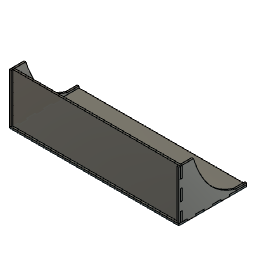
Hilla (Autodesk Fusion 360 design; units mm, degrees)
Autodesk Fusion 360 part; units mm, degrees
sketch "Sketch1" plane through (0, 0, 0) normal (0, 1, 0) x (1, 0, 0)
sketch "Sketch2" plane through (0, 0, 0) normal (0, 1, 0) x (1, 0, 0)
  line L0 (0, 0) -> (500, 0)
  line L1 (500, 0) -> (500, 200)
  line L2 (500, 200) -> (0, 200)
  line L3 (0, 200) -> (0, 0)
  dimension "d5" = 200
  dimension "d6" = 500
  constraint horizontal L0
  constraint vertical L1
  constraint horizontal L2
  constraint vertical L3
  constraint coincident L0.start L3.end
  measures "d5" distance of L0.start L2.end
  measures "d6" distance of L0.start L0.end
extrude "Extrude1" add sketch "Sketch2" along normal blind 5 makes body 1
sketch "Sketch3" plane through (0, 5, 0) normal (0, 1, 0) x (-1, 0, 0)
  line L0 (0, -200) -> (0, 0)
  line L1 (0, 0) -> (-500, 0)
  line L2 (-500, 0) -> (-500, -200)
  line L3 (-500, -200) -> (0, -200)
  line L4 (0, 0) -> (0, -25)
  line L5 (0, -25) -> (-5, -25)
  line L6 (-5, -25) -> (-5, -50)
  line L7 (-5, -50) -> (0, -50)
  line L8 (0, -50) -> (0, -25)
  dimension "d9" = 25
  dimension "d10" = 5
  dimension "d11" = 25
  constraint vertical L4
  constraint coincident L0.end L1.start
  constraint horizontal L5
  constraint vertical L6
  constraint horizontal L7
  constraint vertical L8
  measures "d9" distance of L0.end L4.end
  measures "d10" distance of L4.end L5.end
  measures "d11" distance of L4.end L7.end
extrude "Extrude2" cut sketch "Sketch3" against normal blind 5 contours L0 L5 L6 L7 L8 bodies 1
sketch "Sketch4" plane through (0, 5, 0) normal (0, 1, 0) x (-1, 0, 0)
  line L0 (-5, -25) -> (0, -25)
  line L1 (0, -25) -> (0, 0)
  line L2 (0, 0) -> (-500, 0)
  line L3 (-500, 0) -> (-500, -200)
  line L4 (-500, -200) -> (0, -200)
  line L5 (0, -200) -> (0, -50)
  line L6 (0, -50) -> (-5, -50)
  line L7 (-5, -50) -> (-5, -25)
  line L8 (0, -50) -> (0, -75)
  line L9 (0, -75) -> (-5, -75)
  line L10 (-5, -75) -> (-5, -100)
  line L11 (-5, -100) -> (0, -100)
  line L12 (0, -100) -> (0, -75)
  line L13 (0, -100) -> (0, -125)
  line L14 (0, -125) -> (-5, -125)
  line L15 (-5, -125) -> (-5, -150)
  line L16 (-5, -150) -> (0, -150)
  line L17 (0, -150) -> (0, -125)
  dimension "d14" = 25
  dimension "d15" = 5
  dimension "d16" = 25
  dimension "d17" = 25
  dimension "d18" = 25
  dimension "d19" = 5
  constraint vertical L8
  constraint coincident L5.end L6.start
  constraint horizontal L9
  constraint vertical L10
  constraint horizontal L11
  constraint vertical L12
  constraint vertical L13
  constraint horizontal L14
  constraint vertical L15
  constraint horizontal L16
  constraint vertical L17
  measures "d14" distance of L5.end L8.end
  measures "d15" distance of L8.end L9.end
  measures "d16" distance of L8.end L11.end
  measures "d17" distance of L11.end L13.end
  measures "d18" distance of L13.end L16.end
  measures "d19" distance of L13.end L14.end
extrude "Extrude3" cut sketch "Sketch4" against normal blind 5 contours L5 L9 L10 L11 L12 | L5 L14 L15 L16 L17 bodies 1
sketch "Sketch5" plane through (0, 5, 0) normal (0, 1, 0) x (-1, 0, 0)
  line L0 (0, -150) -> (-5, -150)
  line L1 (-5, -150) -> (-5, -125)
  line L2 (-5, -125) -> (0, -125)
  line L3 (0, -125) -> (0, -100)
  line L4 (0, -100) -> (-5, -100)
  line L5 (-5, -100) -> (-5, -75)
  line L6 (-5, -75) -> (0, -75)
  line L7 (0, -75) -> (0, -50)
  line L8 (0, -50) -> (-5, -50)
  line L9 (-5, -50) -> (-5, -25)
  line L10 (-5, -25) -> (0, -25)
  line L11 (0, -25) -> (0, 0)
  line L12 (0, 0) -> (-500, 0)
  line L13 (-500, 0) -> (-500, -200)
  line L14 (-500, -200) -> (0, -200)
  line L15 (0, -200) -> (0, -150)
  line L16 (-500, 0) -> (-500, -25)
  line L17 (-500, -25) -> (-495, -25)
  line L18 (-495, -25) -> (-495, -50)
  line L19 (-495, -50) -> (-500, -50)
  line L20 (-500, -50) -> (-500, -25)
  line L21 (-500, -50) -> (-500, -37.5)
  line L22 (-500, -37.5) -> (-495, -37.5)
  line L23 (-495, -37.5) -> (-495, -62.5)
  line L24 (-495, -62.5) -> (-500, -62.5)
  line L25 (-500, -62.5) -> (-500, -37.5)
  line L26 (-500, -62.5) -> (-500, -87.5)
  line L27 (-500, -87.5) -> (-495, -87.5)
  line L28 (-495, -87.5) -> (-495, -112.5)
  line L29 (-495, -112.5) -> (-500, -112.5)
  line L30 (-500, -112.5) -> (-500, -87.5)
  dimension "d22" = 25
  dimension "d23" = 5
  dimension "d24" = 25
  dimension "d26" = 25
  dimension "d27" = 5
  dimension "d28" = 25
  dimension "d29" = 25
  dimension "d30" = 5
  constraint vertical L16
  constraint coincident L12.end L13.start
  constraint horizontal L17
  constraint vertical L18
  constraint horizontal L19
  constraint vertical L20
  constraint vertical L21
  constraint horizontal L22
  constraint vertical L23
  constraint horizontal L24
  constraint vertical L25
  constraint vertical L26
  constraint horizontal L27
  constraint vertical L28
  constraint horizontal L29
  constraint vertical L30
  measures "d22" distance of L12.end L16.end
  measures "d23" distance of L16.end L17.end
  measures "d24" distance of L16.end L19.end
  measures "d26" distance of L21.end L24.end
  measures "d27" distance of L21.end L22.end
  measures "d28" distance of L24.end L26.end
  measures "d29" distance of L26.end L29.end
  measures "d30" distance of L26.end L27.end
extrude "Extrude4" cut sketch "Sketch5" against normal blind 5 contours L13 L27 L28 L29 L30 | L13 L19 L23 L24 L25 | L13 L18 L19 L20 L21 L22 L23 L25 | L13 L17 L18 L20 L22 bodies 1
sketch "Sketch6" plane through (0, 5, 0) normal (0, 1, 0) x (-1, 0, 0)
  line L0 (-500, -87.5) -> (-495, -87.5)
  line L1 (-495, -87.5) -> (-495, -112.5)
  line L2 (-500, -62.5) -> (-500, -87.5)
  line L3 (-500, -200) -> (0, -200)
  line L4 (0, -200) -> (0, -150)
  line L5 (0, -150) -> (-5, -150)
  line L6 (-5, -150) -> (-5, -125)
  line L7 (-5, -125) -> (0, -125)
  line L8 (0, -125) -> (0, -100)
  line L9 (0, -100) -> (-5, -100)
  line L10 (-5, -100) -> (-5, -75)
  line L11 (-5, -75) -> (0, -75)
  line L12 (0, -75) -> (0, -50)
  line L13 (0, -50) -> (-5, -50)
  line L14 (-5, -50) -> (-5, -25)
  line L15 (-5, -25) -> (0, -25)
  line L16 (0, -25) -> (0, 0)
  line L17 (0, 0) -> (-500, 0)
  line L18 (-500, 0) -> (-500, -25)
  line L19 (0, 0) -> (0, -5)
  line L20 (0, -5) -> (-60, -5)
  line L21 (-60, -5) -> (-110, -5)
  line L22 (-110, -5) -> (-110, -10)
  line L23 (-110, -10) -> (-60, -10)
  line L24 (-60, -10) -> (-60, -5)
  line L25 (-110, -5) -> (-170, -5)
  line L26 (-170, -5) -> (-220, -5)
  line L27 (-220, -5) -> (-220, -10)
  line L28 (-220, -10) -> (-170, -10)
  line L29 (-170, -10) -> (-170, -5)
  line L30 (-220, -5) -> (-280, -5)
  line L31 (-280, -5) -> (-330, -5)
  line L32 (-330, -5) -> (-330, -10)
  line L33 (-330, -10) -> (-280, -10)
  line L34 (-280, -10) -> (-280, -5)
  line L35 (-330, -5) -> (-390, -5)
  line L36 (-390, -5) -> (-440, -5)
  line L37 (-440, -5) -> (-440, -10)
  line L38 (-440, -10) -> (-390, -10)
  line L39 (-390, -10) -> (-390, -5)
  line L40 (-500, -25) -> (-495, -25)
  line L41 (-495, -25) -> (-495, -62.5)
  line L42 (-495, -62.5) -> (-500, -62.5)
  line L43 (-495, -112.5) -> (-500, -112.5)
  line L44 (-500, -112.5) -> (-500, -200)
  dimension "d33" = 5
  dimension "d34" = 60
  dimension "d35" = 50
  dimension "d36" = 5
  dimension "d37" = 60
  dimension "d38" = 50
  dimension "d39" = 5
  dimension "d40" = 60
  dimension "d41" = 50
  dimension "d42" = 5
  dimension "d43" = 60
  dimension "d44" = 50
  dimension "d45" = 5
  constraint vertical L19
  constraint coincident L16.end L17.start
  constraint horizontal L20
  constraint horizontal L21
  constraint vertical L22
  constraint horizontal L23
  constraint vertical L24
  constraint horizontal L25
  constraint horizontal L26
  constraint vertical L27
  constraint horizontal L28
  constraint vertical L29
  constraint horizontal L30
  constraint horizontal L31
  constraint vertical L32
  constraint horizontal L33
  constraint vertical L34
  constraint horizontal L35
  constraint horizontal L36
  constraint vertical L37
  constraint horizontal L38
  constraint vertical L39
  measures "d33" distance of L16.end L19.end
  measures "d34" distance of L19.end L20.end
  measures "d35" distance of L20.end L21.end
  measures "d36" distance of L20.end L23.end
  measures "d37" distance of L21.end L25.end
  measures "d38" distance of L25.end L26.end
  measures "d39" distance of L25.end L28.end
  measures "d40" distance of L26.end L30.end
  measures "d41" distance of L30.end L31.end
  measures "d42" distance of L30.end L33.end
  measures "d43" distance of L31.end L35.end
  measures "d44" distance of L35.end L36.end
  measures "d45" distance of L35.end L38.end
extrude "Extrude5" cut sketch "Sketch6" against normal blind 5 contours L21 L22 L23 L24 | L26 L27 L28 L29 | L31 L32 L33 L34 | L36 L37 L38 L39 bodies 1
sketch "Sketch7" plane through (0, 0, -10) normal (0, 0, 1) x (1, 0, 0)
  line L0 (110, 5) -> (60, 5)
  line L1 (60, 5) -> (60, 0)
  line L2 (60, 0) -> (110, 0)
  line L3 (110, 0) -> (110, 5)
  line L4 (0, 0) -> (500, 0)
  line L5 (500, 0) -> (500, 150)
  line L6 (500, 150) -> (0, 150)
  line L7 (0, 150) -> (0, 0)
  dimension "d48" = 500
  dimension "d49" = 150
  constraint horizontal L4
  constraint vertical L5
  constraint horizontal L6
  constraint vertical L7
  constraint coincident L4.start L7.end
  measures "d48" distance of L4.start L4.end
  measures "d49" distance of L4.start L6.end
extrude "Extrude6" add sketch "Sketch7" along normal blind 5 separate body contours L0 L1 L3 L4 L5 L6 L7 makes body 2
sketch "Sketch8" plane through (0, 0, 0) normal (-1, 0, 0) x (0, 0, 1)
  line L0 (-10, 150) -> (-10, 0)
  line L1 (-10, 0) -> (-5, 0)
  line L2 (-5, 0) -> (-5, 150)
  line L3 (-5, 150) -> (-10, 150)
  line L4 (-5, 150) -> (-5, 116.6667)
  line L5 (-5, 116.6667) -> (-10, 116.6667)
  line L6 (-10, 116.6667) -> (-10, 91.6667)
  line L7 (-10, 91.6667) -> (-5, 91.6667)
  line L8 (-5, 91.6667) -> (-5, 116.6667)
  line L9 (-5, 91.6667) -> (-5, 58.3333)
  line L10 (-5, 58.3333) -> (-10, 58.3333)
  line L11 (-10, 58.3333) -> (-10, 33.3333)
  line L12 (-10, 33.3333) -> (-5, 33.3333)
  line L13 (-5, 33.3333) -> (-5, 58.3333)
  dimension "d52" = 33.3333
  dimension "d53" = 25
  dimension "d54" = 5
  dimension "d55" = 33.3333
  dimension "d56" = 25
  dimension "d57" = 5
  constraint vertical L4
  constraint coincident L2.end L3.start
  constraint horizontal L5
  constraint vertical L6
  constraint horizontal L7
  constraint vertical L8
  constraint vertical L9
  constraint horizontal L10
  constraint vertical L11
  constraint horizontal L12
  constraint vertical L13
  measures "d52" distance of L2.end L4.end
  measures "d53" distance of L4.end L7.end
  measures "d54" distance of L4.end L5.end
  measures "d55" distance of L7.end L9.end
  measures "d56" distance of L9.end L12.end
  measures "d57" distance of L9.end L10.end
extrude "Extrude7" cut sketch "Sketch8" against normal blind 5 contours L0 L2 L5 L6 L7 L8 | L0 L2 L10 L11 L12 L13 bodies 2
extrude "Extrude8" add 1 faces at (93.3333, 5, -8.3333) along direction (0, -1, 0) blind 5 on bodies 2 bodies 2
combine "Combine1" operation cut target body 2 tool bodies 1 keep tools
sketch "Sketch9" plane through (500, 0, 0) normal (1, 0, 0) x (0, 0, -1)
  line L0 (5, 5) -> (10, 5)
  line L1 (10, 5) -> (10, 150)
  line L2 (10, 150) -> (5, 150)
  line L3 (5, 150) -> (5, 5)
  line L4 (5, 150) -> (5, 116.6667)
  line L5 (5, 116.6667) -> (10, 116.6667)
  line L6 (10, 116.6667) -> (10, 91.6667)
  line L7 (10, 91.6667) -> (5, 91.6667)
  line L8 (5, 91.6667) -> (5, 116.6667)
  line L9 (5, 91.6667) -> (5, 58.3333)
  line L10 (5, 58.3333) -> (10, 58.3333)
  line L11 (10, 58.3333) -> (10, 33.3333)
  line L12 (10, 33.3333) -> (5, 33.3333)
  line L13 (5, 33.3333) -> (5, 58.3333)
  dimension "d62" = 33.3333
  dimension "d63" = 5
  dimension "d64" = 25
  dimension "d65" = 33.3333
  dimension "d66" = 5
  dimension "d67" = 25
  constraint vertical L4
  constraint coincident L2.end L3.start
  constraint horizontal L5
  constraint vertical L6
  constraint horizontal L7
  constraint vertical L8
  constraint vertical L9
  constraint horizontal L10
  constraint vertical L11
  constraint horizontal L12
  constraint vertical L13
  measures "d62" distance of L2.end L4.end
  measures "d63" distance of L4.end L5.end
  measures "d64" distance of L4.end L7.end
  measures "d65" distance of L7.end L9.end
  measures "d66" distance of L9.end L10.end
  measures "d67" distance of L9.end L12.end
extrude "Extrude9" cut sketch "Sketch9" against normal blind 5 contours L1 L3 L10 L11 L12 L13 | L1 L3 L5 L6 L7 L8 bodies 2
sketch "Sketch10" plane through (495, 0, 0) normal (1, 0, 0) x (0, 0, -1)
  line L0 (62.5, 5) -> (25, 5)
  line L1 (25, 0) -> (62.5, 0)
  line L2 (62.5, 0) -> (62.5, 5)
  line L3 (0, 0) -> (200, 0)
  line L4 (200, 0) -> (200, 150)
  line L5 (200, 150) -> (0, 150)
  line L6 (0, 150) -> (0, 0)
  line L7 (62.5, 5) -> (37.5, 5)
  line L8 (37.5, 5) -> (37.5, 0)
  line L9 (37.5, 0) -> (62.5, 0)
  line L10 (62.5, 0) -> (62.5, 5)
  line L11 (25, 5) -> (25, 0)
  dimension "d70" = 200
  dimension "d71" = 150
  dimension "d72" = 25
  dimension "d73" = 5
  constraint horizontal L3
  constraint vertical L4
  constraint horizontal L5
  constraint vertical L6
  constraint coincident L3.start L6.end
  constraint horizontal L7
  constraint vertical L8
  constraint horizontal L9
  constraint vertical L10
  constraint coincident L0.start L2.end
  measures "d70" distance of L3.start L3.end
  measures "d71" distance of L3.start L5.end
  measures "d72" distance of L0.start L7.end
  measures "d73" distance of L0.start L1.end
sketch "Sketch11" plane through (500, 0, 0) normal (1, 0, 0) x (0, 0, -1)
  line L0 (10, 58.3333) -> (5, 58.3333)
  line L1 (5, 58.3333) -> (5, 91.6667)
  line L2 (5, 91.6667) -> (10, 91.6667)
  line L3 (10, 91.6667) -> (10, 58.3333)
  line L4 (5, 5) -> (5, 33.3333)
  line L5 (5, 33.3333) -> (10, 33.3333)
  line L6 (10, 33.3333) -> (10, 5)
  line L7 (10, 5) -> (25, 5)
  line L8 (25, 5) -> (25, 0)
  line L9 (25, 0) -> (62.5, 0)
  line L10 (62.5, 0) -> (62.5, 5)
  line L11 (62.5, 5) -> (87.5, 5)
  line L12 (87.5, 5) -> (87.5, 0)
  line L13 (87.5, 0) -> (112.5, 0)
  line L14 (112.5, 0) -> (112.5, 5)
  line L15 (112.5, 5) -> (200, 5)
  line L16 (200, 5) -> (200, 150)
  line L17 (200, 150) -> (10, 150)
  line L18 (10, 150) -> (10, 116.6667)
  line L19 (10, 116.6667) -> (5, 116.6667)
  line L20 (5, 116.6667) -> (5, 150)
  line L21 (5, 150) -> (0, 150)
  line L22 (0, 150) -> (0, 5)
  line L23 (0, 5) -> (5, 5)
  line L24 (200, 5) -> (200, 10)
  line L25 (200, 10) -> (166.6667, 10)
  line L26 (0, 150) -> (43.3333, 150)
  line L27 (0, 0) -> (94.4755, 54.5455)
  line L28 (0, 0) -> (109.0909, 0) construction
  spline S0 degree 5 poles (43.3333, 150) (44.7384, 145.6171) (47.6386, 136.9857) (52.2594, 124.4419) (58.9705, 108.5369) (68.3404, 90.1184) (78.7871, 73.3054) (90.412, 58.2492) (103.2926, 45.0651) (117.4138, 33.7309) (132.6963, 24.1281) (145.7822, 17.728) (156.0507, 13.605) (163.0949, 11.1523) (166.6667, 10) knots 0 0 0 0 0 0 0.1 0.2 0.3 0.4 0.5 0.6 0.7 0.8 0.9 1 1 1 1 1 1
  dimension "d76" = 5
  dimension "d77" = 33.3333
  dimension "d78" = 43.3333
  dimension "d79" = 30
  dimension "d80" = 109.0909
  constraint vertical L24
  constraint coincident L15.end L16.start
  constraint horizontal L25
  constraint horizontal L26
  constraint coincident L21.end L22.start
  constraint horizontal L28
  constraint coincident L27.start L28.start
  measures "d76" distance of L15.end L24.end
  measures "d77" distance of L24.end L25.end
  measures "d78" distance of L21.end L26.end
  measures "d79" angle of L27 L28
  measures "d80" distance of L27.start L27.end
sketch "Sketch12" plane through (0, 0, 0) normal (-1, 0, 0) x (0, 0, 1)
  line L0 (-125, 5) -> (-125, 0)
  line L1 (-125, 0) -> (-100, 0)
  line L2 (-100, 0) -> (-100, 5)
  line L3 (-100, 5) -> (-125, 5)
  line L4 (0, 0) -> (-200, 0)
  line L5 (-200, 0) -> (-200, 150)
  line L6 (-200, 150) -> (0, 150)
  line L7 (0, 150) -> (0, 0)
  line L8 (-125, 0) -> (-100, 0)
  line L9 (-100, 0) -> (-100, 5)
  line L10 (-100, 5) -> (-125, 5)
  line L11 (-125, 5) -> (-125, 0)
  dimension "d83" = 200
  dimension "d84" = 150
  dimension "d85" = 25
  dimension "d86" = 5
  constraint horizontal L4
  constraint vertical L5
  constraint horizontal L6
  constraint vertical L7
  constraint coincident L4.start L7.end
  constraint horizontal L8
  constraint vertical L9
  constraint horizontal L10
  constraint vertical L11
  constraint coincident L0.end L1.start
  measures "d83" distance of L4.start L4.end
  measures "d84" distance of L4.start L6.end
  measures "d85" distance of L0.end L1.end
  measures "d86" distance of L0.end L0.start
extrude "Extrude12" add sketch "Sketch12" against normal blind 5 separate body makes body 3
combine "Combine4" operation cut target body 3 tool bodies 2 keep tools
combine "Combine5" operation cut target body 3 tool bodies 1 keep tools
sketch "Sketch13" plane through (0, 0, 0) normal (-1, 0, 0) x (0, 0, 1)
  line L0 (-5, 91.6667) -> (-5, 58.3333)
  line L1 (-5, 58.3333) -> (-10, 58.3333)
  line L2 (-10, 58.3333) -> (-10, 91.6667)
  line L3 (-10, 91.6667) -> (-5, 91.6667)
  line L4 (-200, 5) -> (-150, 5)
  line L5 (-150, 5) -> (-150, 0)
  line L6 (-150, 0) -> (-125, 0)
  line L7 (-125, 0) -> (-125, 5)
  line L8 (-125, 5) -> (-100, 5)
  line L9 (-100, 5) -> (-100, 0)
  line L10 (-100, 0) -> (-75, 0)
  line L11 (-75, 0) -> (-75, 5)
  line L12 (-75, 5) -> (-50, 5)
  line L13 (-50, 5) -> (-50, 0)
  line L14 (-50, 0) -> (-25, 0)
  line L15 (-25, 0) -> (-25, 5)
  line L16 (-25, 5) -> (-10, 5)
  line L17 (-10, 5) -> (-10, 33.3333)
  line L18 (-10, 33.3333) -> (-5, 33.3333)
  line L19 (-5, 33.3333) -> (-5, 5)
  line L20 (-5, 5) -> (0, 5)
  line L21 (0, 5) -> (0, 150)
  line L22 (0, 150) -> (-5, 150)
  line L23 (-5, 150) -> (-5, 116.6667)
  line L24 (-5, 116.6667) -> (-10, 116.6667)
  line L25 (-10, 116.6667) -> (-10, 150)
  line L26 (-10, 150) -> (-200, 150)
  line L27 (-200, 150) -> (-200, 5)
  line L28 (-200, 5) -> (-200, 10)
  line L29 (-200, 10) -> (-166.6667, 10)
  line L30 (0, 0) -> (-94.4755, 54.5455)
  line L31 (0, 0) -> (-109.0909, 0) construction
  line L32 (0, 150) -> (-43.3333, 150)
  spline S0 degree 5 poles (-166.6667, 10) (-163.0949, 11.1523) (-156.0507, 13.605) (-145.7822, 17.728) (-132.6963, 24.1281) (-117.4138, 33.7309) (-103.2926, 45.0651) (-90.412, 58.2492) (-78.7871, 73.3054) (-68.3404, 90.1184) (-58.9705, 108.5369) (-52.2594, 124.4419) (-47.6386, 136.9857) (-44.7384, 145.6171) (-43.3333, 150) knots 0 0 0 0 0 0 0.1 0.2 0.3 0.4 0.5 0.6 0.7 0.8 0.9 1 1 1 1 1 1
  dimension "d89" = 5
  dimension "d90" = 33.3333
  dimension "d92" = 30
  dimension "d93" = 109.0909
  dimension "d94" = 43.3333
  constraint vertical L28
  constraint coincident L4.start L27.end
  constraint horizontal L29
  constraint horizontal L31
  constraint coincident L30.start L31.start
  constraint horizontal L32
  constraint coincident L21.end L22.start
  measures "d89" distance of L4.start L28.end
  measures "d90" distance of L28.end L29.end
  measures "d92" angle of L30 L31
  measures "d93" distance of L30.start L30.end
  measures "d94" distance of L21.end L32.end
extrude "Extrude13" cut sketch "Sketch13" against normal blind 5 contours L26 L27 L29 S0 bodies 3
extrude "Extrude14" add 2 faces at (495, 3.3333, -95.8333) (495, 1.6667, -37.5) along direction (1, 0, 0) blind 5 on bodies 1 bodies 1
sketch "Sketch14" plane through (0, 0, 0) normal (0, -1, 0) x (1, 0, 0)
  line L0 (170, -5) -> (220, -5)
  line L1 (220, -5) -> (220, -10)
  line L2 (220, -10) -> (170, -10)
  line L3 (170, -10) -> (170, -5)
  line L4 (280, -5) -> (330, -5)
  line L5 (330, -5) -> (330, -10)
  line L6 (330, -10) -> (280, -10)
  line L7 (280, -10) -> (280, -5)
  line L8 (60, -5) -> (110, -5)
  line L9 (110, -5) -> (110, -10)
  line L10 (110, -10) -> (60, -10)
  line L11 (60, -10) -> (60, -5)
  line L12 (390, -5) -> (440, -5)
  line L13 (440, -5) -> (440, -10)
  line L14 (440, -10) -> (390, -10)
  line L15 (390, -10) -> (390, -5)
  line L16 (500, -200) -> (500, 0)
  line L17 (500, 0) -> (0, 0)
  line L18 (0, 0) -> (0, -25)
  line L19 (0, -25) -> (5, -25)
  line L20 (5, -25) -> (5, -50)
  line L21 (5, -50) -> (0, -50)
  line L22 (0, -50) -> (0, -75)
  line L23 (0, -75) -> (5, -75)
  line L24 (5, -75) -> (5, -100)
  line L25 (5, -100) -> (0, -100)
  line L26 (0, -100) -> (0, -125)
  line L27 (0, -125) -> (5, -125)
  line L28 (5, -125) -> (5, -150)
  line L29 (5, -150) -> (0, -150)
  line L30 (0, -150) -> (0, -200)
  line L31 (0, -200) -> (500, -200)
  line L32 (500, 0) -> (500, -25)
  line L33 (500, -25) -> (495, -25)
  line L34 (495, -25) -> (495, -50)
  line L35 (495, -50) -> (500, -50)
  line L36 (500, -50) -> (500, -25)
  line L37 (500, -50) -> (500, -75)
  line L38 (500, -75) -> (495, -75)
  line L39 (495, -75) -> (495, -100)
  line L40 (495, -100) -> (500, -100)
  line L41 (500, -100) -> (500, -75)
  line L42 (500, -100) -> (500, -125)
  line L43 (500, -125) -> (495, -125)
  line L44 (495, -125) -> (495, -150)
  line L45 (495, -150) -> (500, -150)
  line L46 (500, -150) -> (500, -125)
  dimension "d99" = 25
  dimension "d100" = 25
  dimension "d101" = 5
  dimension "d102" = 25
  dimension "d103" = 5
  dimension "d104" = 25
  dimension "d105" = 25
  dimension "d106" = 25
  dimension "d107" = 5
  constraint vertical L32
  constraint coincident L16.end L17.start
  constraint horizontal L33
  constraint vertical L34
  constraint horizontal L35
  constraint vertical L36
  constraint vertical L37
  constraint horizontal L38
  constraint vertical L39
  constraint horizontal L40
  constraint vertical L41
  constraint vertical L42
  constraint horizontal L43
  constraint vertical L44
  constraint horizontal L45
  constraint vertical L46
  measures "d99" distance of L16.end L32.end
  measures "d100" distance of L32.end L35.end
  measures "d101" distance of L32.end L33.end
  measures "d102" distance of L35.end L37.end
  measures "d103" distance of L37.end L38.end
  measures "d104" distance of L37.end L40.end
  measures "d105" distance of L40.end L42.end
  measures "d106" distance of L42.end L45.end
  measures "d107" distance of L42.end L43.end
extrude "Extrude15" cut sketch "Sketch14" against normal blind 5 contours L16 L43 L44 L45 L46 | L16 L38 L39 L40 L41 | L16 L33 L34 L35 L36 bodies 1
sketch "Sketch15" plane through (0, 0, 0) normal (0, -1, 0) x (1, 0, 0)
  line L0 (500, -150) -> (495, -150)
  line L1 (495, -150) -> (495, -125)
  line L2 (495, -125) -> (500, -125)
  line L3 (500, -125) -> (500, -100)
  line L4 (500, -100) -> (495, -100)
  line L5 (495, -100) -> (495, -75)
  line L6 (495, -75) -> (500, -75)
  line L7 (500, -75) -> (500, -50)
  line L8 (500, -50) -> (495, -50)
  line L9 (495, -50) -> (495, -25)
  line L10 (495, -25) -> (500, -25)
  line L11 (500, -25) -> (500, 0)
  line L12 (500, 0) -> (0, 0)
  line L13 (0, 0) -> (0, -25)
  line L14 (0, -25) -> (5, -25)
  line L15 (5, -25) -> (5, -50)
  line L16 (5, -50) -> (0, -50)
  line L17 (0, -50) -> (0, -75)
  line L18 (0, -75) -> (5, -75)
  line L19 (5, -75) -> (5, -100)
  line L20 (5, -100) -> (0, -100)
  line L21 (0, -100) -> (0, -125)
  line L22 (0, -125) -> (5, -125)
  line L23 (5, -125) -> (5, -150)
  line L24 (5, -150) -> (0, -150)
  line L25 (0, -150) -> (0, -200)
  line L26 (0, -200) -> (500, -200)
  line L27 (500, -200) -> (500, -150)
  line L28 (390, -5) -> (440, -5)
  line L29 (440, -5) -> (440, -10)
  line L30 (440, -10) -> (390, -10)
  line L31 (390, -10) -> (390, -5)
  line L32 (60, -5) -> (110, -5)
  line L33 (110, -5) -> (110, -10)
  line L34 (110, -10) -> (60, -10)
  line L35 (60, -10) -> (60, -5)
  line L36 (280, -5) -> (330, -5)
  line L37 (330, -5) -> (330, -10)
  line L38 (330, -10) -> (280, -10)
  line L39 (280, -10) -> (280, -5)
  line L40 (170, -5) -> (220, -5)
  line L41 (220, -5) -> (220, -10)
  line L42 (220, -10) -> (170, -10)
  line L43 (170, -10) -> (170, -5)
sketch "Sketch16" plane through (495, 0, 0) normal (1, 0, 0) x (0, 0, -1)
  line L0 (75, 0) -> (100, 0)
  line L1 (100, 0) -> (100, 5)
  line L2 (100, 5) -> (75, 5)
  line L3 (75, 5) -> (75, 0)
  line L4 (0, 0) -> (200, 0)
  line L5 (200, 0) -> (200, 150)
  line L6 (200, 150) -> (0, 150)
  line L7 (0, 150) -> (0, 0)
  line L8 (75, 5) -> (100, 5)
  line L9 (100, 5) -> (100, 0)
  line L10 (100, 0) -> (75, 0)
  line L11 (75, 0) -> (75, 5)
  dimension "d110" = 200
  dimension "d111" = 150
  dimension "d112" = 25
  dimension "d113" = 5
  constraint horizontal L4
  constraint vertical L5
  constraint horizontal L6
  constraint vertical L7
  constraint coincident L4.start L7.end
  constraint horizontal L8
  constraint vertical L9
  constraint horizontal L10
  constraint vertical L11
  constraint coincident L2.end L3.start
  measures "d110" distance of L4.start L4.end
  measures "d111" distance of L4.start L6.end
  measures "d112" distance of L2.end L1.end
  measures "d113" distance of L2.end L0.start
extrude "Extrude16" add sketch "Sketch16" along normal blind 5 separate body makes body 4
combine "Combine6" operation cut target body 4 tool bodies 2 keep tools
combine "Combine7" operation cut target body 4 tool bodies 2 keep tools
combine "Combine8" operation cut target body 4 tool bodies 1 keep tools
sketch "Sketch17" plane through (500, 0, 0) normal (1, 0, 0) x (0, 0, -1)
  line L0 (150, 5) -> (200, 5)
  line L1 (200, 5) -> (200, 150)
  line L2 (200, 150) -> (10, 150)
  line L3 (10, 150) -> (10, 116.6667)
  line L4 (10, 116.6667) -> (5, 116.6667)
  line L5 (5, 116.6667) -> (5, 150)
  line L6 (5, 150) -> (0, 150)
  line L7 (0, 150) -> (0, 5)
  line L8 (0, 5) -> (5, 5)
  line L9 (5, 5) -> (5, 33.3333)
  line L10 (5, 33.3333) -> (10, 33.3333)
  line L11 (10, 33.3333) -> (10, 5)
  line L12 (10, 5) -> (25, 5)
  line L13 (25, 5) -> (25, 0)
  line L14 (25, 0) -> (50, 0)
  line L15 (50, 0) -> (50, 5)
  line L16 (50, 5) -> (75, 5)
  line L17 (75, 5) -> (75, 0)
  line L18 (75, 0) -> (100, 0)
  line L19 (100, 0) -> (100, 5)
  line L20 (100, 5) -> (125, 5)
  line L21 (125, 5) -> (125, 0)
  line L22 (125, 0) -> (150, 0)
  line L23 (150, 0) -> (150, 5)
  line L24 (10, 58.3333) -> (5, 58.3333)
  line L25 (5, 58.3333) -> (5, 91.6667)
  line L26 (5, 91.6667) -> (10, 91.6667)
  line L27 (10, 91.6667) -> (10, 58.3333)
  line L28 (0, 150) -> (43.3333, 150)
  line L29 (200, 5) -> (200, 10)
  line L30 (200, 10) -> (166.6667, 10)
  line L31 (0, 0) -> (94.4755, 54.5455)
  line L32 (0, 0) -> (109.0909, 0) construction
  spline S0 degree 5 poles (43.3333, 150) (44.7384, 145.6171) (47.6386, 136.9857) (52.2594, 124.4419) (58.9705, 108.5369) (68.3404, 90.1184) (78.7871, 73.3054) (90.412, 58.2492) (103.2926, 45.0651) (117.4138, 33.7309) (132.6963, 24.1281) (145.7822, 17.728) (156.0507, 13.605) (163.0949, 11.1523) (166.6667, 10) knots 0 0 0 0 0 0 0.1 0.2 0.3 0.4 0.5 0.6 0.7 0.8 0.9 1 1 1 1 1 1
  dimension "d116" = 43.3333
  dimension "d117" = 5
  dimension "d118" = 33.3333
  dimension "d119" = 30
  dimension "d120" = 109.0909
  constraint horizontal L28
  constraint coincident L6.end L7.start
  constraint vertical L29
  constraint coincident L0.end L1.start
  constraint horizontal L30
  constraint horizontal L32
  constraint coincident L31.start L32.start
  measures "d116" distance of L6.end L28.end
  measures "d117" distance of L0.end L29.end
  measures "d118" distance of L29.end L30.end
  measures "d119" angle of L31 L32
  measures "d120" distance of L31.start L31.end
extrude "Extrude17" cut sketch "Sketch17" against normal blind 5 contours L1 L2 L30 S0 bodies 4
equation "haed = 200 mm"
equation "breidd = 500 mm"
equation "Thykkt = 5 mm"
equation "Dypt = 150 mm"
equation "d5 = haed"
equation "d6 = breidd"
equation "d7 = Thykkt"
equation "d9 = haed * ( 1 / 8 )"
equation "d10 = Thykkt"
equation "d11 = haed * ( 1 / 8 )"
equation "d12 = -Thykkt"
equation "d14 = haed * ( 1 / 8 )"
equation "d15 = Thykkt"
equation "d16 = haed * ( 1 / 8 )"
equation "d17 = haed * ( 1 / 8 )"
equation "d18 = haed * ( 1 / 8 )"
equation "d19 = Thykkt"
equation "d20 = -Thykkt"
equation "d22 = haed * ( 1 / 8 )"
equation "d23 = Thykkt"
equation "d24 = haed * ( 1 / 8 )"
equation "d25 = haed * ( 1 / 8 )"
equation "d26 = haed * ( 1 / 8 )"
equation "d27 = Thykkt"
equation "d28 = haed * ( 1 / 8 )"
equation "d29 = haed * ( 1 / 8 )"
equation "d30 = Thykkt"
equation "d31 = -Thykkt"
equation "d33 = Thykkt"
equation "d34 = breidd * ( 60 / 500 )"
equation "d35 = breidd * ( 50 / 500 )"
equation "d36 = Thykkt"
equation "d37 = breidd * ( 60 / 500 )"
equation "d38 = breidd * ( 50 / 500 )"
equation "d39 = Thykkt"
equation "d40 = breidd * ( 60 / 500 )"
equation "d41 = breidd * ( 50 / 500 )"
equation "d42 = Thykkt"
equation "d43 = breidd * ( 60 / 500 )"
equation "d44 = breidd * ( 50 / 500 )"
equation "d45 = Thykkt"
equation "d46 = -Thykkt"
equation "d48 = breidd"
equation "d49 = Dypt"
equation "d50 = Thykkt"
equation "d52 = Dypt * ( 100 / 450 )"
equation "d53 = Dypt * ( 25 / 150 )"
equation "d54 = Thykkt"
equation "d55 = Dypt * ( 100 / 450 )"
equation "d56 = Dypt * ( 25 / 150 )"
equation "d57 = Thykkt"
equation "d58 = -Thykkt"
equation "d60 = Thykkt"
equation "d62 = Dypt * ( 100 / 450 )"
equation "d63 = Thykkt"
equation "d64 = Dypt * ( 25 / 150 )"
equation "d65 = Dypt * ( 100 / 450 )"
equation "d66 = Thykkt"
equation "d67 = Dypt * ( 25 / 150 )"
equation "d68 = -Thykkt"
equation "d70 = haed"
equation "d71 = Dypt"
equation "d72 = haed * ( 25 / 200 )"
equation "d73 = Thykkt"
equation "d76 = Thykkt"
equation "d77 = haed * ( 1 / 6 )"
equation "d78 = Thykkt * 2 + haed * ( 1 / 6 )"
equation "d80 = haed * ( 6 / 11 )"
equation "d83 = haed"
equation "d84 = Dypt"
equation "d85 = haed * ( 25 / 200 )"
equation "d86 = Thykkt"
equation "d87 = -Thykkt"
equation "d89 = Thykkt"
equation "d90 = haed * ( 1 / 6 )"
equation "d93 = haed * ( 6 / 11 )"
equation "d94 = Thykkt * 2 + haed * ( 1 / 6 )"
equation "d95 = -Thykkt"
equation "d97 = Thykkt"
equation "d99 = haed * ( 1 / 8 )"
equation "d100 = haed * ( 1 / 8 )"
equation "d101 = Thykkt"
equation "d102 = haed * ( 1 / 8 )"
equation "d103 = Thykkt"
equation "d104 = haed * ( 1 / 8 )"
equation "d105 = haed * ( 1 / 8 )"
equation "d106 = haed * ( 1 / 8 )"
equation "d107 = Thykkt"
equation "d108 = -Thykkt"
equation "d110 = haed"
equation "d111 = Dypt"
equation "d112 = haed * ( 1 / 8 )"
equation "d114 = Thykkt"
equation "d116 = 2 * Thykkt + haed * ( 1 / 6 )"
equation "d117 = Thykkt"
equation "d118 = haed * ( 1 / 6 )"
equation "d120 = haed * ( 6 / 11 )"
equation "d121 = -Thykkt"
